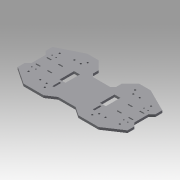
# Autodesk Inventor part: Support_Moteur
Saved by Autodesk Inventor 2016 (Build 200138000, 138)
## iProperties
Created: 2015-09-29
Part Number: Support_Moteur
Material: Générique
Document SubType Name: Modeling
Designer: Logan
Density: 1 g/cm^3
Appearance: Par défaut
Author: Logan
Autodesk Inventor part; units mm, degrees
ref_plane "YZ Plane" through (0, 0, 0) normal (1, 0, 0) x (0, 1, 0)
ref_plane "XZ Plane" through (0, 0, 0) normal (0, 1, 0) x (-1, 0, 0)
ref_plane "XY Plane" through (0, 0, 0) normal (0, 0, 1) x (1, 0, 0)
sketch "Esquisse1" plane through (0, 0, 0) normal (0, 0, 1) x (1, 0, 0)
  line L0 (-190, -60) -> (-190, 60)
  line L1 (190, 60) -> (190, -60)
  line L2 (-110, 100) -> (-190, 60)
  line L3 (110, 100) -> (190, 60)
  line L4 (-190, -60) -> (-130, -100)
  line L5 (130, -100) -> (190, -60)
  line L6 (70, 100) -> (110, 100)
  line L7 (130, -100) -> (60, -100)
  line L8 (-60, -100) -> (-130, -100)
  line L9 (30, 40) -> (-30, 40)
  line L10 (-110, 100) -> (-70, 100)
  line L11 (60, 100) -> (110, 100)
  line L12 (-60, -100) -> (-30, -80)
  line L13 (-30, -80) -> (30, -80)
  line L14 (30, -80) -> (60, -100)
  line L15 (-40, 50) -> (-40, 70)
  line L16 (40, 50) -> (40, 70)
  line L17 (-30, 40) -> (-40, 50)
  line L18 (30, 40) -> (40, 50)
  line L19 (-70, 100) -> (-40, 70)
  line L20 (70, 100) -> (40, 70)
  point P0 (0, 0)
  point P1 (-60, 100)
  point P2 (-40, 40)
  point P3 (40, 40)
  point P4 (-40, 100)
  point P5 (40, 100)
  dimension "d204" = 60
  dimension "d207" = 40
  dimension "d208" = 40
  dimension "d211" = 20
  dimension "d212" = 30
  dimension "d213" = 30
  dimension "d214" = 10
  dimension "d215" = 10
  dimension "d216" = 10
  dimension "d217" = 10
  dimension "d218" = 30
  dimension "d219" = 30
  dimension "d220" = 30
  dimension "d221" = 30
  dimension "d227" = 80
  dimension "d228" = 40
  dimension "d229" = 60
  dimension "d230" = 40
  dimension "d231" = 80
  dimension "d232" = 40
  dimension "d233" = 60
  dimension "d234" = 380
  dimension "d235" = 190
  dimension "d236" = 30
  dimension "d250" = 60
  dimension "d251" = 40
  constraints: 42 end point, 10 point on line, 7 parallel, 3 horizontal, 2 collinear, 2 perpendicular, 2 vertical
  measures "d204" distance between parallel lines of L9 L10
  measures "d207" horizontal distance of point (0, 0) point (40, 40)
  measures "d208" horizontal distance of point (0, 0) point (-40, 40)
  measures "d211" distance between parallel lines of L8 L13
  measures "d212" horizontal distance of L12.end L8.start
  measures "d213" horizontal distance of L7.end L13.end
  measures "d214" distance of L9.end point (-40, 40)
  measures "d215" distance of L15.start point (-40, 40)
  measures "d216" distance of L9.start point (40, 40)
  measures "d217" distance of L16.start point (40, 40)
  measures "d218" distance of L10.end point (-40, 100)
  measures "d219" distance of L15.end point (-40, 100)
  measures "d220" distance of L6.start point (40, 100)
  measures "d221" distance of L16.end point (40, 100)
  measures "d227" horizontal distance of L2.start L0.end
  measures "d228" vertical distance of L2.start L0.end
  measures "d229" horizontal distance of L0.start L4.end
  measures "d230" vertical distance of L0.start L4.end
  measures "d231" horizontal distance of L3.start L1.start
  measures "d232" vertical distance of L3.start L1.start
  measures "d233" distance of L12.end L13.end
  measures "d234" distance between parallel lines of L1 L0
  measures "d235" distance from line of point (0, 0) L0
  measures "d236" horizontal distance of point (0, 0) L13.end
  measures "d250" horizontal distance of L5.start L1.end
  measures "d251" vertical distance of L5.start L1.end
extrude "Plaque" add sketch "Esquisse1" along normal blind 8
sketch "Esquisse2" plane through (0, 0, 8) normal (0, 0, 1) x (1, 0, 0)
  circle A0 centre (-166, 35) radius 2
  circle A1 centre (-152, 35) radius 2
  circle A2 centre (-166, -35) radius 2
  circle A3 centre (-152, -35) radius 2
  line L0 (-190, 60) -> (-190, -60) projected
  line L1 (0, 25.5561) -> (0, -26.1527)
  circle A4 centre (166, 35) radius 2
  circle A5 centre (152, 35) radius 2
  circle A6 centre (166, -35) radius 2
  circle A7 centre (152, -35) radius 2
  point P0 (0, 0)
  dimension "d12" = 4
  dimension "d13" = 4
  dimension "d14" = 4
  dimension "d15" = 4
  dimension "d16" = 14
  dimension "d17" = 14
  dimension "d18" = 24
  dimension "d19" = 24
  dimension "d20" = 35
  dimension "d21" = 35
  dimension "d22" = 35
  dimension "d23" = 35
  constraints: 8 centre point, 4 symmetric about line, 2 end point, 1 vertical, 4 other
  measures "d12" diameter of A0
  measures "d13" diameter of A1
  measures "d14" diameter of A3
  measures "d15" diameter of A2
  measures "d16" distance of A1.centre A0.centre
  measures "d17" distance of A3.centre A2.centre
  measures "d18" distance from line of L0 A0.centre
  measures "d19" distance from line of L0 A2.centre
  measures "d20" vertical distance of point (0, 0) A2.centre
  measures "d21" vertical distance of point (0, 0) A3.centre
  measures "d22" vertical distance of point (0, 0) A1.centre
  measures "d23" vertical distance of point (0, 0) A0.centre
hole "Fixation_Encodeur" at (-152, 35, 8) at (-166, 35, 8) at (-166, -35, 8) at (-152, -35, 8) at (152, 35, 8) at (166, 35, 8) at (166, -35, 8) at (152, -35, 8) direction (0, 0, -1) diameter 4 end through all
sketch "Esquisse3" plane through (0, 0, 8) normal (0, 0, 1) x (1, 0, 0)
  line L0 (-120.5, -19) -> (-120.5, 19)
  line L1 (-160.5, 19) -> (-160.5, -19)
  line L2 (-160.5, -19) -> (-120.5, 19) construction
  line L3 (-120.5, -19) -> (-160.5, 19) construction
  line L4 (-110, 100) -> (-190, 60) projected
  line L5 (-190, 60) -> (-190, -60) projected
  line L6 (-190, -60) -> (-130, -100) projected
  line L7 (60, -100) -> (130, -100) projected
  line L8 (130, -100) -> (190, -60) projected
  line L9 (190, -60) -> (190, 60) projected
  line L10 (190, 60) -> (110, 100) projected
  line L11 (-70, 100) -> (-110, 100) projected
  line L12 (0, 102.1518) -> (0, -90)
  line L13 (-130, -100) -> (-60, -100) projected
  line L14 (30, 40) -> (-30, 40) projected
  line L15 (-60, -100) -> (-30, -80) projected
  line L16 (-30, -80) -> (30, -80) projected
  line L17 (30, -80) -> (60, -100) projected
  line L18 (70, 100) -> (40, 70) projected
  line L19 (40, 70) -> (40, 50) projected
  line L20 (40, 50) -> (30, 40) projected
  line L21 (-30, 40) -> (-40, 50) projected
  line L22 (-40, 50) -> (-40, 70) projected
  line L23 (-40, 70) -> (-70, 100) projected
  line L24 (110, 100) -> (70, 100) projected
  line L25 (-166.5, 19) -> (-154.5, 19)
  line L26 (-126.5, 19) -> (-114.5, 19)
  line L27 (-30, 0) -> (30, 0)
  line L28 (-166.5, 19) -> (-154.5, 19) construction
  line L29 (-166.5, 17) -> (-154.5, 17)
  line L30 (-154.5, 21) -> (-166.5, 21)
  arc A0 (-166.5, 21) -> (-166.5, 17) centre (-166.5, 19) ccw
  arc A1 (-154.5, 17) -> (-154.5, 21) centre (-154.5, 19) ccw
  line L31 (-126.5, 19) -> (-114.5, 19) construction
  line L32 (-126.5, 17) -> (-114.5, 17)
  line L33 (-114.5, 21) -> (-126.5, 21)
  arc A2 (-126.5, 21) -> (-126.5, 17) centre (-126.5, 19) ccw
  arc A3 (-114.5, 17) -> (-114.5, 21) centre (-114.5, 19) ccw
  line L34 (-166.5, -19) -> (-154.5, -19)
  line L35 (-126.5, -19) -> (-114.5, -19)
  line L36 (-166.5, -19) -> (-154.5, -19) construction
  line L37 (-166.5, -17) -> (-154.5, -17)
  line L38 (-154.5, -21) -> (-166.5, -21)
  arc A4 (-166.5, -17) -> (-166.5, -21) centre (-166.5, -19) ccw
  arc A5 (-154.5, -21) -> (-154.5, -17) centre (-154.5, -19) ccw
  line L39 (-126.5, -19) -> (-114.5, -19) construction
  line L40 (-126.5, -17) -> (-114.5, -17)
  line L41 (-114.5, -21) -> (-126.5, -21)
  arc A6 (-126.5, -17) -> (-126.5, -21) centre (-126.5, -19) ccw
  arc A7 (-114.5, -21) -> (-114.5, -17) centre (-114.5, -19) ccw
  line L42 (120.5, -19) -> (120.5, 19)
  line L43 (160.5, 19) -> (160.5, -19)
  line L44 (160.5, -19) -> (120.5, 19) construction
  line L45 (120.5, -19) -> (160.5, 19) construction
  line L46 (166.5, 19) -> (154.5, 19)
  line L47 (126.5, 19) -> (114.5, 19)
  line L48 (166.5, 19) -> (154.5, 19) construction
  line L49 (166.5, 17) -> (154.5, 17)
  line L50 (154.5, 21) -> (166.5, 21)
  arc A8 (166.5, 17) -> (166.5, 21) centre (166.5, 19) ccw
  arc A9 (154.5, 21) -> (154.5, 17) centre (154.5, 19) ccw
  line L51 (126.5, 19) -> (114.5, 19) construction
  line L52 (126.5, 17) -> (114.5, 17)
  line L53 (114.5, 21) -> (126.5, 21)
  arc A10 (126.5, 17) -> (126.5, 21) centre (126.5, 19) ccw
  arc A11 (114.5, 21) -> (114.5, 17) centre (114.5, 19) ccw
  arc A12 (154.5, -17) -> (154.5, -21) centre (154.5, -19) ccw
  line L54 (166.5, -19) -> (154.5, -19) construction
  line L55 (166.5, -19) -> (154.5, -19)
  line L56 (166.5, -17) -> (154.5, -17)
  arc A13 (166.5, -21) -> (166.5, -17) centre (166.5, -19) ccw
  line L57 (114.5, -21) -> (126.5, -21)
  line L58 (154.5, -21) -> (166.5, -21)
  line L59 (126.5, -17) -> (114.5, -17)
  line L60 (126.5, -19) -> (114.5, -19)
  line L61 (126.5, -19) -> (114.5, -19) construction
  arc A14 (114.5, -17) -> (114.5, -21) centre (114.5, -19) ccw
  arc A15 (126.5, -21) -> (126.5, -17) centre (126.5, -19) ccw
  point P0 (0, 0)
  point P1 (-140.5, 0)
  point P2 (-120.5, 19)
  point P3 (-160.5, -19)
  point P4 (-120.5, -19)
  point P5 (140.5, 0)
  point P6 (120.5, 19)
  point P7 (160.5, -19)
  point P8 (120.5, -19)
  dimension "d31" = 29.5
  dimension "d32" = 40
  dimension "d242" = 12
  dimension "d243" = 6
  dimension "d244" = 12
  dimension "d245" = 6
  dimension "d246" = 4
  dimension "d247" = 4
  constraints: 100 end point, 47 symmetric about line, 32 point on circle, 16 centre point, 14 midpoint, 8 tangent, 5 equal length, 2 horizontal, 1 vertical, 12 other
  measures "d31" distance between parallel lines of L5 L1
  measures "d32" distance between parallel lines of L1 L0
  measures "d242" distance of L25.start L25.end
  measures "d243" distance from line of L25.start L1
  measures "d244" distance of L26.start L26.end
  measures "d245" distance from line of L0 L26.end
  measures "d246" diameter of A1
  measures "d247" diameter of A3
extrude "Extrusion5" cut sketch "Esquisse3" against normal up to next contours A0 L30 A1 L29 | A2 L33 A3 L32 | L37 A5 L38 A4 | L40 A7 L41 A6 | L49 A9 L50 A8 | L52 A11 L53 A10 | L56 A13 L58 A12 | A14 L59 A15 L57
sketch "Esquisse4" plane through (0, 0, 8) normal (0, 0, 1) x (1, 0, 0)
  line L0 (-80, -25) -> (-60, -25)
  line L1 (-80, 25) -> (-80, -25)
  line L2 (-80, -25) -> (-59.915, 7.067) construction
  line L3 (-110, 100) -> (-190, 60) projected
  line L4 (-190, 60) -> (-190, -60) projected
  line L5 (-190, -60) -> (-130, -100) projected
  line L6 (60, -100) -> (130, -100) projected
  line L7 (130, -100) -> (190, -60) projected
  line L8 (190, -60) -> (190, 60) projected
  line L9 (190, 60) -> (110, 100) projected
  line L10 (-70, 100) -> (-110, 100) projected
  line L11 (60, 25) -> (80, 25)
  line L12 (80, 25) -> (80, -25)
  line L13 (80, -25) -> (60, -10.6364) construction
  line L14 (60, 25) -> (60, -25)
  line L15 (-60, -25) -> (-60, 25)
  line L16 (-60, 25) -> (-80, 25)
  line L17 (-59.915, 7.067) -> (-80, 25) construction
  line L18 (60, 10.0232) -> (80, 25) construction
  line L19 (80, -25) -> (60, -25)
  line L20 (-130, -100) -> (-60, -100) projected
  line L21 (30, 40) -> (-30, 40) projected
  line L22 (-60, -100) -> (-30, -80) projected
  line L23 (-30, -80) -> (30, -80) projected
  line L24 (30, -80) -> (60, -100) projected
  line L25 (70, 100) -> (40, 70) projected
  line L26 (40, 70) -> (40, 50) projected
  line L27 (40, 50) -> (30, 40) projected
  line L28 (-30, 40) -> (-40, 50) projected
  line L29 (-40, 50) -> (-40, 70) projected
  line L30 (-40, 70) -> (-70, 100) projected
  line L31 (110, 100) -> (70, 100) projected
  point P0 (-59.915, 7.067)
  dimension "d50" = 110
  dimension "d157" = 110
  dimension "d158" = 20
  dimension "d159" = 20
  constraints: 24 end point, 3 point on line, 2 collinear, 2 parallel, 1 horizontal
  measures "d50" distance between parallel lines of L4 L1
  measures "d157" distance between parallel lines of L8 L12
  measures "d158" distance between parallel lines of L1 L15
  measures "d159" distance between parallel lines of L12 L14
extrude "Passage_Courroie" cut sketch "Esquisse4" against normal up to surface (8 mm away) contours L1 L16 L15 L0 | L11 L12 L19 L14
sketch "Esquisse5" plane through (0, 0, 8) normal (0, 0, 1) x (1, 0, 0)
  line L0 (0, 30.4597) -> (0, -30.4597)
  line L1 (-17.5456, 0) -> (17.5456, 0)
  line L2 (-158, 53.1115) -> (-116.2229, 74)
  line L3 (-116.2229, 74) -> (-82, 74)
  line L4 (-82, 74) -> (-82, -74)
  line L5 (-82, -74) -> (-129.1054, -74)
  line L6 (-129.1054, -74) -> (-158, -54.4961)
  line L7 (116.2229, 74) -> (82, 74)
  line L8 (158, 53.1115) -> (116.2229, 74)
  line L9 (82, -74) -> (129.1054, -74)
  line L10 (129.1054, -74) -> (158, -54.4961)
  line L11 (-190, 60) -> (-190, -60) projected
  point P0 (0, 0)
  point P1 (0, 0)
  dimension "d175" = 47.1054
  dimension "d176" = 34.2229
  dimension "d177" = 41.7771
  dimension "d178" = 28.8946
  dimension "d179" = 32
  dimension "d180" = 32
  dimension "d240" = 148
  constraints: 22 end point, 6 symmetric about line, 2 midpoint, 2 vertical, 1 coincident, 1 horizontal
  measures "d175" distance of L4.end L5.end
  measures "d176" distance of L3.start L3.end
  measures "d177" horizontal distance of L2.start L3.start
  measures "d178" horizontal distance of L5.end L6.end
  measures "d179" distance from line of L11 L6.end
  measures "d180" distance from line of L11 L2.start
  measures "d240" distance of L3.end L4.end
hole "Fixation_Base" at (158, 53.1115, 8) at (82, 74, 8) at (158, -54.4961, 8) at (82, -74, 8) at (-82, -74, 8) at (-158, -54.4961, 8) at (-158, 53.1115, 8) at (-82, 74, 8) direction (0, 0, -1) diameter 6 end through all
sketch "Esquisse8" plane through (0, 0, 8) normal (0, 0, 1) x (1, 0, 0)
  line L0 (-178, -30) -> (-190, -30)
  line L1 (-190, -30) -> (-190, 30)
  line L2 (-190, 30) -> (-178, 30)
  line L3 (-178, 30) -> (-178, -30)
  line L4 (-178, -30) -> (-190, 30) construction
  line L5 (-190, -30) -> (-178, 30) construction
  line L6 (0, 43.7993) -> (0, -83.0015)
  line L7 (178, -30) -> (190, -30)
  line L8 (190, -30) -> (190, 30)
  line L9 (190, 30) -> (178, 30)
  line L10 (178, 30) -> (178, -30)
  line L11 (178, -30) -> (190, 30) construction
  line L12 (190, -30) -> (178, 30) construction
  point P0 (0, 0)
  point P1 (-184, 0)
  point P2 (184, 0)
  dimension "d106" = 60
  dimension "d107" = 12
  dimension "d108" = 178
  dimension "d191" = 30
  constraints: 26 end point, 5 symmetric about line, 4 midpoint, 2 parallel, 1 horizontal, 1 perpendicular, 1 vertical
  measures "d106" distance of L2.end L0.start
  measures "d107" distance of L1.end L2.end
  measures "d108" distance from line of point (0, 0) L3
  measures "d191" distance from line of point (0, 0) L2
extrude "Passage_Encodeur" cut sketch "Esquisse8" against normal up to surface (8 mm away)
chamfer "Chanfrein1" distance 6 angle 45 8 edges at (-178, 30, 4) (-178, -30, 4) (178, 30, 4) (178, -30, 4) (190, 30, 4) (-190, 30, 4) (-190, -30, 4) (190, -30, 4)
sketch "Esquisse10" plane through (0, 0, 8) normal (0, 0, 1) x (1, 0, 0)
  line L0 (-70, -35) -> (-70, -55) construction
  line L1 (-73, -35) -> (-73, -55)
  line L2 (-67, -55) -> (-67, -35)
  arc A0 (-67, -35) -> (-73, -35) centre (-70, -35) ccw
  arc A1 (-73, -55) -> (-67, -55) centre (-70, -55) ccw
  line L3 (-60, -25) -> (-80, -25) projected
  line L4 (0, 0) -> (0, -51.7085)
  line L5 (70, -35) -> (70, -55) construction
  line L6 (73, -35) -> (73, -55)
  line L7 (67, -55) -> (67, -35)
  arc A2 (73, -35) -> (67, -35) centre (70, -35) ccw
  arc A3 (67, -55) -> (73, -55) centre (70, -55) ccw
  point P0 (-70, -45)
  point P1 (70, -45)
  dimension "d192" = 10
  dimension "d193" = 20
  dimension "d194" = 3
  dimension "d195" = 10
  constraints: 18 end point, 8 point on circle, 7 symmetric about line, 4 centre point, 4 tangent, 2 vertical, 1 midpoint, 1 parallel, 2 other
  measures "d192" distance from line of L3 L0.start
  measures "d193" distance of L0.start L0.end
  measures "d194" distance from line of point (-70, -45) L2
  measures "d195" horizontal distance of L3.end point (-70, -45)
extrude "Extrusion4" cut sketch "Esquisse10" against normal blind 10
sketch "Esquisse11" plane through (0, 0, 8) normal (0, 0, 1) x (1, 0, 0)
  line L0 (0, 0) -> (0, -70.3583)
  line L1 (-113, 59) -> (-91, 59)
  line L2 (-91, 59) -> (-91, -59)
  line L3 (-91, -59) -> (-113, -59)
  line L4 (-113, -59) -> (-113, 59)
  line L5 (-80, -25) -> (-80, 25) projected
  line L6 (113, 59) -> (91, 59)
  line L7 (91, 59) -> (91, -59)
  line L8 (91, -59) -> (113, -59)
  line L9 (113, -59) -> (113, 59)
  dimension "d252" = 118
  dimension "d253" = 59
  dimension "d254" = 22
  dimension "d255" = 11
  constraints: 18 end point, 4 symmetric about line, 2 parallel, 1 horizontal, 1 perpendicular, 1 vertical
  measures "d252" distance between parallel lines of L3 L1
  measures "d253" distance from line of L0.start L3
  measures "d254" distance between parallel lines of L2 L4
  measures "d255" distance between parallel lines of L5 L2
hole "Perçage7" at (-113, 59, 8) at (-91, 59, 8) at (-113, -59, 8) at (-91, -59, 8) at (91, -59, 8) at (113, -59, 8) at (113, 59, 8) at (91, 59, 8) direction (0, 0, -1) diameter 6 end through all
